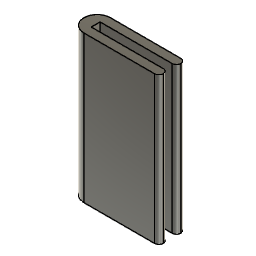
jointer (Autodesk Fusion 360 design; units mm, degrees)
part number: 2025-07-04-23-09-59-403
Autodesk Fusion 360 part; units mm, degrees
sketch "Schizzo1" plane through (0, 0, 0) normal (0, 0, 1) x (1, 0, 0)
  line L0 (0, 0) -> (10, 0)
  line L1 (10, 0) -> (10, 2)
  line L2 (10, 2) -> (0, 2)
  line L3 (0, 2) -> (0, 0)
  line L4 (0, 2) -> (2.5, 2)
  line L5 (2.5, 2) -> (2.5, 4)
  line L6 (2.5, 4) -> (0, 4)
  line L7 (0, 4) -> (0, 2)
  line L8 (0, 4) -> (10, 4)
  line L9 (10, 4) -> (10, 6)
  line L10 (10, 6) -> (0, 6)
  line L11 (0, 6) -> (0, 4)
  dimension "d1" = 10
  dimension "d2" = 2
  dimension "d3" = 2
  constraint horizontal L0
  constraint vertical L1
  constraint horizontal L2
  constraint vertical L3
  constraint coincident L0.start L3.end
  constraint horizontal L4
  constraint vertical L5
  constraint horizontal L6
  constraint vertical L7
  constraint horizontal L8
  constraint vertical L9
  constraint horizontal L10
  constraint vertical L11
  measures "d1" distance of L0.start L0.end
  measures "d2" distance of L0.start L2.end
  measures "d3" distance of L2.end L6.end
sketch "Schizzo2" plane through (0, 0, 0) normal (0, 0, 1) x (1, 0, 0)
  line L0 (0, 0) -> (30, 0)
  line L1 (30, 0) -> (30, 3)
  line L2 (30, 3) -> (0, 3)
  line L3 (0, 3) -> (0, 0)
  line L4 (0, 3) -> (10, 3)
  line L5 (10, 3) -> (10, 6)
  line L6 (10, 6) -> (0, 6)
  line L7 (0, 6) -> (0, 3)
  line L8 (0, 6) -> (30, 6)
  line L9 (30, 6) -> (30, 9)
  line L10 (30, 9) -> (0, 9)
  line L11 (0, 9) -> (0, 6)
  constraint horizontal L0
  constraint vertical L1
  constraint horizontal L2
  constraint vertical L3
  constraint coincident L0.start L3.end
  constraint horizontal L4
  constraint vertical L5
  constraint horizontal L6
  constraint vertical L7
  constraint horizontal L8
  constraint vertical L9
  constraint horizontal L10
  constraint vertical L11
extrude "Estrusione2" add sketch "Schizzo2" along normal blind 50
fillet "Raccordo3" radius 4.5 2 edges at (0, 0, 25) (0, 9, 25)
fillet "Raccordo4" radius 1.5 4 edges at (30, 0, 25) (30, 3, 25) (30, 6, 25) (30, 9, 25)
extrude "Estrusione3" cut 1 faces at (10, 4, 33.3333) along direction (-1, 0, 0) blind 6
extrude "Estrusione1" [suppressed]
fillet "Raccordo1" [suppressed]
fillet "Raccordo2" [suppressed]
